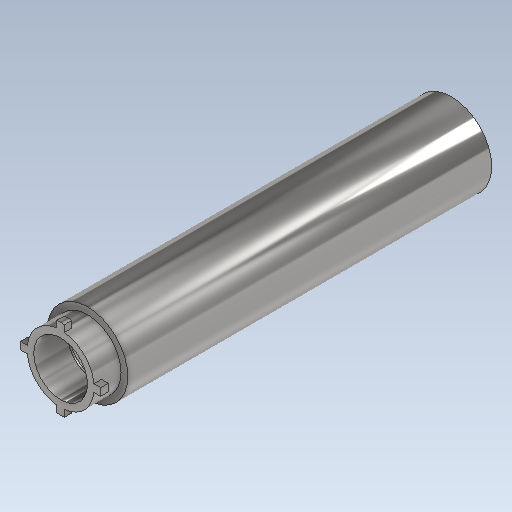
# Autodesk Inventor part: HERRAMIENTA_p2
Saved by Autodesk Inventor 2026 (Build 300175000, 175)
## iProperties
Created: 2026-07-16
Part Number: HERRAMIENTA_p2
Material: Plástico PET
Document SubType Name: Sheet Metal
Designer: User
Density: 1.541 g/cm^3
Sheet Metal Rule: Por defecto_mm
Appearance: Acero - Pulido
Author: User
Autodesk Inventor part; units mm, degrees
ref_plane "YZ Plane" through (0, 0, 0) normal (1, 0, 0) x (0, 1, 0)
ref_plane "XZ Plane" through (0, 0, 0) normal (0, 1, 0) x (-1, 0, 0)
ref_plane "XY Plane" through (0, 0, 0) normal (0, 0, 1) x (1, 0, 0)
sketch "Boceto1" plane through (0, 0, 0) normal (0, 0, 1) x (1, 0, 0)
  circle A0 centre (0, 0) radius 15
  dimension "d0" = 30
  constraints: 1 centre point, 1 coincident
  measures "d0" diameter of A0
extrude "Extrusión1" add sketch "Boceto1" along normal blind 145.5
sketch "Boceto2" plane through (0, 0, 145.5) normal (0, 0, 1) x (1, 0, 0)
  circle A0 centre (0, 0) radius 12.5
  circle A1 centre (0, 0) radius 15
  dimension "d5" = 25
  constraints: 2 centre point, 1 coincident
  measures "d5" diameter of A0
extrude "Extrusión2" cut sketch "Boceto2" against normal blind 10
sketch "Boceto3" plane through (0, 0, 145.5) normal (0, 0, 1) x (1, 0, 0)
  circle A0 centre (0, 0) radius 10
  dimension "d8" = 20
  constraints: 1 centre point, 1 coincident
  measures "d8" diameter of A0
extrude "Extrusión3" cut sketch "Boceto3" against normal blind 145.5
sketch "Boceto4" plane through (0, 0, 145.5) normal (0, 0, 1) x (1, 0, 0)
  circle A0 centre (0, 0) radius 15
  circle A1 centre (0, 0) radius 12.5 projected
  line L0 (-14.9345, 1.4) -> (-12.4214, 1.4)
  line L1 (-12.4214, 1.4) -> (-12.4214, -1.4)
  line L2 (-12.4214, -1.4) -> (-14.9345, -1.4)
  line L3 (-15.0786, 1.4) -> (-12.4214, -1.4) construction
  line L4 (-12.4214, 1.4) -> (-14.9469, -1.2612) construction
  line L5 (-1.4, -14.9345) -> (-1.4, -12.4214)
  line L6 (-1.4, -12.4214) -> (1.4, -12.4214)
  line L7 (1.4, -12.4214) -> (1.4, -14.9345)
  line L8 (-1.4, -15.0786) -> (1.4, -12.4214) construction
  line L9 (-1.4, -12.4214) -> (1.2612, -14.9469) construction
  line L10 (14.9345, -1.4) -> (12.4214, -1.4)
  line L11 (12.4214, -1.4) -> (12.4214, 1.4)
  line L12 (12.4214, 1.4) -> (14.9345, 1.4)
  line L13 (15.0786, -1.4) -> (12.4214, 1.4) construction
  line L14 (12.4214, -1.4) -> (14.9469, 1.2612) construction
  line L15 (1.4, 14.9345) -> (1.4, 12.4214)
  line L16 (1.4, 12.4214) -> (-1.4, 12.4214)
  line L17 (-1.4, 12.4214) -> (-1.4, 14.9345)
  line L18 (1.4, 15.0786) -> (-1.4, 12.4214) construction
  line L19 (1.4, 12.4214) -> (-1.2612, 14.9469) construction
  point P0 (-13.75, 0)
  point P1 (0, -13.75)
  point P2 (13.75, 0)
  point P3 (0, 13.75)
  dimension "d12" = 2.8
  dimension "d15" = 360
  constraints: 40 end point, 4 point on line, 3 point on circle, 1 centre point, 1 coincident, 1 horizontal, 1 midpoint, 1 parallel, 1 perpendicular, 51 other
  measures "d12" distance of L0.end L1.end
extrude "Extrusión4" add sketch "Boceto4" against normal blind 2.8 contours A0 L10 A1 L12 | L15 A1 L17 A0 | A0 L5 A1 L7 | L0 A1 L2 A0
sketch "Boceto5" plane through (0, 0, 0) normal (0, 0, -1) x (-1, 0, 0)
  circle A0 centre (0, 0) radius 12.5
  circle A1 centre (0, 0) radius 10
  constraints: 2 centre point, 2 coincident
extrude "Extrusión5" cut sketch "Boceto5" against normal blind 133
fillet "Empalme1" radius 2.5 1 edges at (12.5, 0, 133)
sketch "Boceto6" plane through (0, 0, 0) normal (0, 0, -1) x (-1, 0, 0)
  circle A0 centre (0, 0) radius 12.5 projected
  circle A1 centre (0, 0) radius 12.5
  circle A2 centre (0, 0) radius 10.925
  dimension "d22" = 21.85
  constraints: 2 centre point, 2 coincident
  measures "d22" diameter of A2
extrude "Extrusión6" add sketch "Boceto6" against normal blind 5
equation "\"Radio_pliegue\" = Grosor"
equation "\"Anchura_desahogo_plegado\" = Grosor"
equation "\"Profundidad_desahogo_plegado\" = 0.5 * Grosor"
equation "\"Tamaño_destalonado\" = 4 * Grosor"
equation "\"Remanente_mínimo\" = 2 * Grosor"
equation "\"Radiodetransición\" = Radio_pliegue"
equation "\"Tamaño_de_radio_de_Jacobi\" = Radio_pliegue"
equation "\"TamañoSeparación\" = Grosor"
equation "\"Grosor\" = 0.5"
